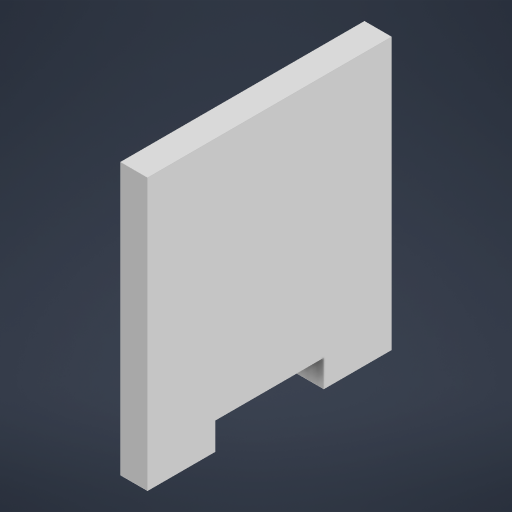
# Autodesk Inventor part: Langbektang houder
Saved by Autodesk Inventor 2023.2 (Build 272271000, 271)
## iProperties
Created: 2020-09-09
Part Number: Langbektang houder
Material: Generic
Document SubType Name: Modeling
Designer: nathan.bollaert
Density: 1 g/cm^3
Appearance: Default
Author: nathan.bollaert
Autodesk Inventor part; units mm, degrees
ref_plane "YZ Plane" through (0, 0, 0) normal (1, 0, 0) x (0, 1, 0)
ref_plane "XZ Plane" through (0, 0, 0) normal (0, 1, 0) x (-1, 0, 0)
ref_plane "XY Plane" through (0, 0, 0) normal (0, 0, 1) x (1, 0, 0)
sketch "Sketch1" plane through (0, 0, 0) normal (1, 0, 0) x (0, 1, 0)
  line L0 (0, 0) -> (-4, 0)
  line L1 (-4, 0) -> (-4, -36)
  line L2 (-4, -36) -> (0, -36)
  line L3 (0, -36) -> (0, 0)
  line L4 (0, -10) -> (-4, -10)
  line L5 (0, -26) -> (-4, -26)
  line L6 (0, 0) -> (36, 0)
  line L7 (36, 0) -> (36, -36)
  line L8 (36, -36) -> (0, -36)
  line L9 (0, -36) -> (0, 0)
  dimension "d228" = 4
  dimension "d229" = 36
  dimension "d230" = 36
  dimension "d231" = 36
  dimension "d232" = 10
  dimension "d233" = 10
  constraints: 20 end point, 4 parallel, 4 perpendicular, 4 point on line, 2 horizontal, 1 coincident
  measures "d228" distance of L2.end L1.end
  measures "d229" distance of L1.end L0.end
  measures "d230" distance of L7.end L8.end
  measures "d231" distance of L6.end L7.end
  measures "d232" distance between parallel lines of L0 L4
  measures "d233" distance between parallel lines of L2 L5
extrude "Extrusion1" add sketch "Sketch1" against normal blind 4 contours L3 L4 L1 L0 | L6 L7 L8 L3 | L3 L2 L1 L5
body "Solid5"
